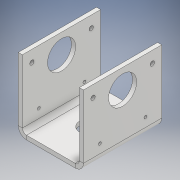
# Autodesk Inventor part: Ground_Tracker_Bearing
Saved by Autodesk Inventor 2018 (Build 220112000, 112)
## iProperties
Created: 2018-09-27
Part Number: Ground_Tracker_Bearing
Material: UHMW, White
Document SubType Name: Sheet Metal
Designer: Bradley
Density: 0.94 g/cm^3
Sheet Metal Rule: Default_mm
Appearance: Smooth - White
Mass: 155.888 g
Surface Area: 601.623 cm^2
Volume: 165.839 cm^3
Author: Bradley
Autodesk Inventor part; units mm, degrees
ref_plane "YZ Plane" through (0, 0, 0) normal (1, 0, 0) x (0, 1, 0)
ref_plane "XZ Plane" through (0, 0, 0) normal (0, 1, 0) x (-1, 0, 0)
ref_plane "XY Plane" through (0, 0, 0) normal (0, 0, 1) x (1, 0, 0)
sketch "Sketch1" plane through (0, 0, 0) normal (0, 0, 1) x (1, 0, 0)
  line L0 (-50, -60) -> (50, -60)
  line L1 (50, -60) -> (50, 60)
  line L2 (50, 60) -> (-50, 60)
  line L3 (-50, 60) -> (-50, -60)
  line L4 (-50, -60) -> (50, 60) construction
  line L5 (50, -60) -> (-50, 60) construction
  point P0 (0, 0)
  dimension "d0" = 100
  dimension "d1" = 120
  measures "d0" distance of L2.end L1.end
  measures "d1" distance of L1.end L0.end
extrude "Plate1" add sketch "Sketch1" along normal blind 6.35
sketch "Sketch2" plane through (-43.65, -60, 0) normal (-1, 0, 0) x (0, -1, 0)
  line L0 (-120, 0) -> (0, 0)
  line L1 (0, 0) -> (0, 110)
  line L2 (0, 110) -> (-120, 110)
  line L3 (-120, 110) -> (-120, 0)
  constraints: 6 end point, 1 horizontal, 1 perpendicular, 1 vertical
edge flange "Flange1" height 110 angle 90 thickness 6.35 bend radius 6.35 thickness toward (-1, 0, 0) relief tear relief width 6.35 relief depth 3.175 corner gap 6.35 corner form 0 edges at (-50, 0, 6.35) (50, 0, 6.35) wall of the first edge with corners at (-43.65, 60, 0) (-43.65, -60, 0) (-43.65, -60, 110) (-43.65, 60, 110)
bend "Bend1"
corner "Corner1"
sketch "Sketch3" plane through (50, -60, 110) normal (1, 0, 0) x (0, 0, -1)
  circle A0 centre (30, 60) radius 21.082 construction
  circle A1 centre (30, 60) radius 21.5
  point P0 (110, 60)
  dimension "d13" = 42.164
  dimension "d14" = 43
  dimension "d15" = 80
  constraints: 2 centre point, 1 coincident, 1 horizontal alignment
  measures "d13" diameter of A0
  measures "d14" diameter of A1
  measures "d15" distance of point (110, 60) A0.centre
extrude "Cut1" cut sketch "Sketch3" against normal through all
sketch "Sketch4" plane through (0, 0, 6.35) normal (0, 0, 1) x (1, 0, 0)
  circle A0 centre (0, 0) radius 15.5
  dimension "d18" = 31
  constraints: 1 centre point, 1 coincident
  measures "d18" diameter of A0
extrude "Cut2" cut sketch "Sketch4" against normal blind 6.35
sketch "Sketch5" plane through (50, -60, 110) normal (1, 0, 0) x (0, 0, -1)
  circle A0 centre (30, 60) radius 21.5 projected
  line L0 (97.3, 0) -> (97.3, 120) projected
  line L1 (0, 120) -> (97.3, 120) projected
  line L2 (0, 0) -> (0, 120) projected
  line L3 (97.3, 0) -> (0, 0) projected
  line L4 (0, 120) -> (97.3, 120) construction
  line L5 (97.3, 0) -> (0, 0) construction
  line L6 (17.542, 105.5) -> (17.542, 14.5) construction
  line L7 (0, 0) -> (0, 120) construction
  point P0 (110, 60)
  point P1 (0, 60)
  point P2 (17.542, 60)
  dimension "d38" = 17.542
  dimension "d39" = 45.5
  constraints: 2 end point, 2 midpoint, 1 horizontal alignment, 1 vertical
  measures "d38" distance between parallel lines of L2 L6
  measures "d39" distance of point (17.542, 60) L6.end
hole "Hole1" at (50, -45.5, 92.458) at (50, 45.5, 92.458) direction (-1, 0, 0) diameter 6.6 end through all clearance for "Flat Head Machine Screw" size "M6" standard "Ansi Metric M Profile"
sketch "Sketch6" plane through (50, -60, 110) normal (1, 0, 0) x (0, 0, -1)
  circle A0 centre (17.542, 14.5) radius 3.3 projected
  circle A1 centre (17.542, 105.5) radius 3.3 projected
  circle A2 centre (30, 60) radius 21.5 projected
  line L0 (97.3, 0) -> (97.3, 120) projected
  line L1 (0, 120) -> (97.3, 120) projected
  line L2 (0, 0) -> (0, 120) projected
  line L3 (97.3, 0) -> (0, 0) projected
  line L4 (83.542, 25) -> (83.542, 95) construction
  point P0 (110, 60)
  point P1 (83.542, 60)
  dimension "d29" = 70
  dimension "d30" = 83.542
  constraints: 2 coincident, 2 end point, 1 horizontal alignment, 1 midpoint, 1 vertical
  measures "d29" distance of L4.start L4.end
  measures "d30" distance between parallel lines of L4 L2
hole "Hole2" at (50, -35, 26.458) at (50, 35, 26.458) direction (-1, 0, 0) diameter 4.5 end through all clearance for "Flat Head Machine Screw" size "M4" standard "Ansi Metric M Profile"
equation "\"d16\" = Thickness"
equation "\"d19\" = Thickness"
equation "\"d27\" = Thickness"
equation "\"d36\" = Thickness"
equation "\"d2\" = Thickness"
equation "\"d3\" = BendReliefWidth"
equation "\"d4\" = BendReliefDepth"
equation "\"d5\" = MinimumRemnant"
equation "\"d6\" = TransitionRadius"
equation "\"d9\" = BendRadius"
equation "\"d10\" = CornerReliefSize"
equation "\"d11\" = GapSize"
equation "\"d12\" = JacobiRadiusSize"
equation "\"BendRadius\" = Thickness"
equation "\"BendReliefWidth\" = Thickness"
equation "\"BendReliefDepth\" = 0.5 * Thickness"
equation "\"CornerReliefSize\" = 4 * Thickness"
equation "\"MinimumRemnant\" = 2 * Thickness"
equation "\"TransitionRadius\" = BendRadius"
equation "\"JacobiRadiusSize\" = BendRadius"
equation "\"GapSize\" = Thickness"
equation "\"Thickness\" = 6.35"
body "Solid1"
